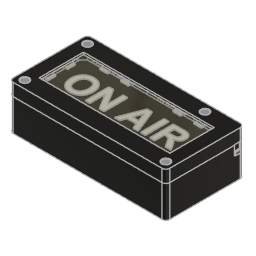
little-on-air-v2 (Autodesk Fusion 360 design; units mm, degrees)
description: Front face down; removable optics; shared left/bottom datums
description: Laser only; rear-engrave mirrored shared vector master
description: 1.6 mm black; 0.4 mm white letters; integral hidden spacer pads
description: Flat frame down, LED pads up; no electronics mounts
description: Optional 1.6 mm laminate only; omit with printed backing; print 0.1 mm layers
description: Rear face down; integral nests, ports, controls and blind M3 bosses
description: Front face down, contact legs up; use M3x8 button heads
description: Flat-sided golf tee; broad flat side down; positive 0.5 mm travel stop
description: Socket end down; 45 degree expanding shoulder; grip passes through wall
description: 52x21x10 pouch; foam and wiring not modeled
description: Provisional bare PCB, USB and component envelopes
description: 21x17.8 board; reset and populated envelopes remain provisional
description: Updated actuator dimensions; throw interpreted from slot length
description: 8x8x2; emitter offset assumed 1 mm
description: 4x25 socket head, 2x6 button head, 2x8 button head
description: Eight standard 5.5 AF x 2.4 mm nuts
Autodesk Fusion 360 part; units mm, degrees
(part 1 of 5)
sketch "Front bezel envelope profile" plane through (0, 0, 0) normal (0, 0, 1) x (1, 0, 0) in component "01 Front optical bezel"
  line L0 (3, 0) -> (117, 0)
  line L1 (120, 3) -> (120, 57)
  line L2 (117, 60) -> (3, 60)
  line L3 (0, 57) -> (0, 3)
  arc A0 (117, 0) -> (120, 3) centre (117, 3) ccw
  arc A1 (120, 57) -> (117, 60) centre (117, 57) ccw
  arc A2 (3, 60) -> (0, 57) centre (3, 57) ccw
  arc A3 (0, 3) -> (3, 0) centre (3, 3) ccw
extrude "Front bezel envelope" add sketch "Front bezel envelope profile" against normal blind 9.5 makes body 1 in component "01 Front optical bezel"
ref_plane "WorkPlane1" through (0, 0, -1.6) normal (0, 0, 1) x (1, 0, 0) in component "01 Front optical bezel"
sketch "Rear open cavity profile" plane through (0, 0, -1.6) normal (0, 0, 1) x (1, 0, 0) in component "01 Front optical bezel"
  line L0 (2.4, 2.4) -> (117.6, 2.4)
  line L1 (117.6, 2.4) -> (117.6, 57.6)
  line L2 (117.6, 57.6) -> (2.4, 57.6)
  line L3 (2.4, 57.6) -> (2.4, 2.4)
  dimension "d39" = 115.2
  dimension "d40" = 55.2
  measures "d39" horizontal distance of L0.start L0.end
  measures "d40" vertical distance of L0.end L1.end
extrude "Rear open cavity" cut sketch "Rear open cavity profile" against normal blind 8 bodies 1 in component "01 Front optical bezel"
ref_plane "WorkPlane2" through (0, 0, 0.02) normal (0, 0, 1) x (1, 0, 0) in component "01 Front optical bezel"
sketch "Visible optical window profile" plane through (0, 0, 0.02) normal (0, 0, 1) x (1, 0, 0) in component "01 Front optical bezel"
  line L0 (10, 13) -> (110, 13)
  line L1 (110, 13) -> (110, 47)
  line L2 (110, 47) -> (10, 47)
  line L3 (10, 47) -> (10, 13)
  dimension "d45" = 100
  dimension "d46" = 34
  measures "d45" horizontal distance of L0.start L0.end
  measures "d46" vertical distance of L0.end L1.end
extrude "Visible optical window" cut sketch "Visible optical window profile" against normal blind 1.64 bodies 1 in component "01 Front optical bezel"
ref_plane "WorkPlane3" through (0, 0, -1.5) normal (0, 0, 1) x (1, 0, 0) in component "01 Front optical bezel"
sketch "Front compression seat profile" plane through (0, 0, -1.5) normal (0, 0, 1) x (1, 0, 0) in component "01 Front optical bezel"
  line L0 (1.8, 1.8) -> (10.2, 1.8)
  line L1 (10.2, 1.8) -> (10.2, 10.2)
  line L2 (10.2, 10.2) -> (1.8, 10.2)
  line L3 (1.8, 10.2) -> (1.8, 1.8)
  dimension "d51" = 8.4
  dimension "d52" = 8.4
  measures "d51" horizontal distance of L0.start L0.end
  measures "d52" vertical distance of L0.end L1.end
extrude "Front compression seat" add sketch "Front compression seat profile" against normal blind 8 separate body makes body 2 in component "01 Front optical bezel"
ref_plane "WorkPlane4" through (0, 0, -1.5) normal (0, 0, 1) x (1, 0, 0) in component "01 Front optical bezel"
sketch "Front compression seat profile (1)" plane through (0, 0, -1.5) normal (0, 0, 1) x (1, 0, 0) in component "01 Front optical bezel"
  line L0 (109.8, 1.8) -> (118.2, 1.8)
  line L1 (118.2, 1.8) -> (118.2, 10.2)
  line L2 (118.2, 10.2) -> (109.8, 10.2)
  line L3 (109.8, 10.2) -> (109.8, 1.8)
  dimension "d57" = 8.4
  dimension "d58" = 8.4
  measures "d57" horizontal distance of L0.start L0.end
  measures "d58" vertical distance of L0.end L1.end
extrude "Front compression seat (1)" add sketch "Front compression seat profile (1)" against normal blind 8 separate body makes body 3 in component "01 Front optical bezel"
ref_plane "WorkPlane5" through (0, 0, -1.5) normal (0, 0, 1) x (1, 0, 0) in component "01 Front optical bezel"
sketch "Front compression seat profile (2)" plane through (0, 0, -1.5) normal (0, 0, 1) x (1, 0, 0) in component "01 Front optical bezel"
  line L0 (1.8, 49.8) -> (10.2, 49.8)
  line L1 (10.2, 49.8) -> (10.2, 58.2)
  line L2 (10.2, 58.2) -> (1.8, 58.2)
  line L3 (1.8, 58.2) -> (1.8, 49.8)
  dimension "d63" = 8.4
  dimension "d64" = 8.4
  measures "d63" horizontal distance of L0.start L0.end
  measures "d64" vertical distance of L0.end L1.end
extrude "Front compression seat (2)" add sketch "Front compression seat profile (2)" against normal blind 8 separate body makes body 4 in component "01 Front optical bezel"
ref_plane "WorkPlane6" through (0, 0, -1.5) normal (0, 0, 1) x (1, 0, 0) in component "01 Front optical bezel"
sketch "Front compression seat profile (3)" plane through (0, 0, -1.5) normal (0, 0, 1) x (1, 0, 0) in component "01 Front optical bezel"
  line L0 (91.8, 49.8) -> (100.2, 49.8)
  line L1 (100.2, 49.8) -> (100.2, 58.2)
  line L2 (100.2, 58.2) -> (91.8, 58.2)
  line L3 (91.8, 58.2) -> (91.8, 49.8)
  dimension "d69" = 8.4
  dimension "d70" = 8.4
  measures "d69" horizontal distance of L0.start L0.end
  measures "d70" vertical distance of L0.end L1.end
extrude "Front compression seat (3)" add sketch "Front compression seat profile (3)" against normal blind 8 separate body makes body 5 in component "01 Front optical bezel"
combine "Union manufactured solid" operation add target body 1 tool bodies 2 3 4 5 in component "01 Front optical bezel"
ref_plane "WorkPlane7" through (0, 0, 0.02) normal (0, 0, 1) x (1, 0, 0) in component "01 Front optical bezel"
sketch "M3 through clearance profile" plane through (0, 0, 0.02) normal (0, 0, 1) x (1, 0, 0) in component "01 Front optical bezel"
  circle A0 centre (6, 6) radius 1.7
  dimension "d75" = 3.4
  measures "d75" diameter of A0
extrude "M3 through clearance" cut sketch "M3 through clearance profile" against normal blind 9.6 bodies 1 in component "01 Front optical bezel"
ref_plane "WorkPlane8" through (0, 0, 0.02) normal (0, 0, 1) x (1, 0, 0) in component "01 Front optical bezel"
sketch "Recessed socket head profile" plane through (0, 0, 0.02) normal (0, 0, 1) x (1, 0, 0) in component "01 Front optical bezel"
  circle A0 centre (6, 6) radius 3.2
  dimension "d80" = 6.4
  measures "d80" diameter of A0
extrude "Recessed socket head" cut sketch "Recessed socket head profile" against normal blind 3.22 bodies 1 in component "01 Front optical bezel"
ref_plane "WorkPlane9" through (0, 0, 0.02) normal (0, 0, 1) x (1, 0, 0) in component "01 Front optical bezel"
sketch "M3 through clearance profile (1)" plane through (0, 0, 0.02) normal (0, 0, 1) x (1, 0, 0) in component "01 Front optical bezel"
  circle A0 centre (114, 6) radius 1.7
  dimension "d85" = 3.4
  measures "d85" diameter of A0
extrude "M3 through clearance (1)" cut sketch "M3 through clearance profile (1)" against normal blind 9.6 bodies 1 in component "01 Front optical bezel"
ref_plane "WorkPlane10" through (0, 0, 0.02) normal (0, 0, 1) x (1, 0, 0) in component "01 Front optical bezel"
sketch "Recessed socket head profile (1)" plane through (0, 0, 0.02) normal (0, 0, 1) x (1, 0, 0) in component "01 Front optical bezel"
  circle A0 centre (114, 6) radius 3.2
  dimension "d90" = 6.4
  measures "d90" diameter of A0
extrude "Recessed socket head (1)" cut sketch "Recessed socket head profile (1)" against normal blind 3.22 bodies 1 in component "01 Front optical bezel"
ref_plane "WorkPlane11" through (0, 0, 0.02) normal (0, 0, 1) x (1, 0, 0) in component "01 Front optical bezel"
sketch "M3 through clearance profile (2)" plane through (0, 0, 0.02) normal (0, 0, 1) x (1, 0, 0) in component "01 Front optical bezel"
  circle A0 centre (6, 54) radius 1.7
  dimension "d95" = 3.4
  measures "d95" diameter of A0
extrude "M3 through clearance (2)" cut sketch "M3 through clearance profile (2)" against normal blind 9.6 bodies 1 in component "01 Front optical bezel"
ref_plane "WorkPlane12" through (0, 0, 0.02) normal (0, 0, 1) x (1, 0, 0) in component "01 Front optical bezel"
sketch "Recessed socket head profile (2)" plane through (0, 0, 0.02) normal (0, 0, 1) x (1, 0, 0) in component "01 Front optical bezel"
  circle A0 centre (6, 54) radius 3.2
  dimension "d100" = 6.4
  measures "d100" diameter of A0
extrude "Recessed socket head (2)" cut sketch "Recessed socket head profile (2)" against normal blind 3.22 bodies 1 in component "01 Front optical bezel"
ref_plane "WorkPlane13" through (0, 0, 0.02) normal (0, 0, 1) x (1, 0, 0) in component "01 Front optical bezel"
sketch "M3 through clearance profile (3)" plane through (0, 0, 0.02) normal (0, 0, 1) x (1, 0, 0) in component "01 Front optical bezel"
  circle A0 centre (96, 54) radius 1.7
  dimension "d105" = 3.4
  measures "d105" diameter of A0
extrude "M3 through clearance (3)" cut sketch "M3 through clearance profile (3)" against normal blind 9.6 bodies 1 in component "01 Front optical bezel"
ref_plane "WorkPlane14" through (0, 0, 0.02) normal (0, 0, 1) x (1, 0, 0) in component "01 Front optical bezel"
sketch "Recessed socket head profile (3)" plane through (0, 0, 0.02) normal (0, 0, 1) x (1, 0, 0) in component "01 Front optical bezel"
  circle A0 centre (96, 54) radius 3.2
  dimension "d110" = 6.4
  measures "d110" diameter of A0
extrude "Recessed socket head (3)" cut sketch "Recessed socket head profile (3)" against normal blind 3.22 bodies 1 in component "01 Front optical bezel"
ref_plane "WorkPlane15" through (0, 0, -1.5) normal (0, 0, 1) x (1, 0, 0) in component "01 Front optical bezel"
sketch "LED floor profile" plane through (0, 0, -1.5) normal (0, 0, 1) x (1, 0, 0) in component "01 Front optical bezel"
  line L0 (35.7, 2.4) -> (44.3, 2.4)
  line L1 (44.3, 2.4) -> (44.3, 11.2)
  line L2 (44.3, 11.2) -> (35.7, 11.2)
  line L3 (35.7, 11.2) -> (35.7, 2.4)
  dimension "d115" = 8.6
  dimension "d116" = 8.8
  measures "d115" horizontal distance of L0.start L0.end
  measures "d116" vertical distance of L0.end L1.end
extrude "LED floor" add sketch "LED floor profile" against normal blind 0.6875 separate body makes body 6 in component "01 Front optical bezel"
ref_plane "WorkPlane16" through (0, 0, -1.5) normal (0, 0, 1) x (1, 0, 0) in component "01 Front optical bezel"
sketch "LED lateral guide profile" plane through (0, 0, -1.5) normal (0, 0, 1) x (1, 0, 0) in component "01 Front optical bezel"
  line L0 (34.5, 2.4) -> (35.75, 2.4)
  line L1 (35.75, 2.4) -> (35.75, 11.2)
  line L2 (35.75, 11.2) -> (34.5, 11.2)
  line L3 (34.5, 11.2) -> (34.5, 2.4)
  dimension "d121" = 1.25
  dimension "d122" = 8.8
  measures "d121" horizontal distance of L0.start L0.end
  measures "d122" vertical distance of L0.end L1.end
extrude "LED lateral guide" add sketch "LED lateral guide profile" against normal blind 3 separate body makes body 7 in component "01 Front optical bezel"
ref_plane "WorkPlane17" through (0, 0, -1.5) normal (0, 0, 1) x (1, 0, 0) in component "01 Front optical bezel"
sketch "LED lateral guide profile (1)" plane through (0, 0, -1.5) normal (0, 0, 1) x (1, 0, 0) in component "01 Front optical bezel"
  line L0 (44.25, 2.4) -> (45.5, 2.4)
  line L1 (45.5, 2.4) -> (45.5, 11.2)
  line L2 (45.5, 11.2) -> (44.25, 11.2)
  line L3 (44.25, 11.2) -> (44.25, 2.4)
  dimension "d127" = 1.25
  dimension "d128" = 8.8
  measures "d127" horizontal distance of L0.start L0.end
  measures "d128" vertical distance of L0.end L1.end
extrude "LED lateral guide (1)" add sketch "LED lateral guide profile (1)" against normal blind 3 separate body makes body 8 in component "01 Front optical bezel"
ref_plane "WorkPlane18" through (0, 0, -1.5) normal (0, 0, 1) x (1, 0, 0) in component "01 Front optical bezel"
sketch "LED floor profile (1)" plane through (0, 0, -1.5) normal (0, 0, 1) x (1, 0, 0) in component "01 Front optical bezel"
  line L0 (35.7, 48.8) -> (44.3, 48.8)
  line L1 (44.3, 48.8) -> (44.3, 57.6)
  line L2 (44.3, 57.6) -> (35.7, 57.6)
  line L3 (35.7, 57.6) -> (35.7, 48.8)
  dimension "d133" = 8.6
  dimension "d134" = 8.8
  measures "d133" horizontal distance of L0.start L0.end
  measures "d134" vertical distance of L0.end L1.end
extrude "LED floor (1)" add sketch "LED floor profile (1)" against normal blind 0.6875 separate body makes body 9 in component "01 Front optical bezel"
ref_plane "WorkPlane19" through (0, 0, -1.5) normal (0, 0, 1) x (1, 0, 0) in component "01 Front optical bezel"
sketch "LED lateral guide profile (2)" plane through (0, 0, -1.5) normal (0, 0, 1) x (1, 0, 0) in component "01 Front optical bezel"
  line L0 (34.5, 48.8) -> (35.75, 48.8)
  line L1 (35.75, 48.8) -> (35.75, 57.6)
  line L2 (35.75, 57.6) -> (34.5, 57.6)
  line L3 (34.5, 57.6) -> (34.5, 48.8)
  dimension "d139" = 1.25
  dimension "d140" = 8.8
  measures "d139" horizontal distance of L0.start L0.end
  measures "d140" vertical distance of L0.end L1.end
extrude "LED lateral guide (2)" add sketch "LED lateral guide profile (2)" against normal blind 3 separate body makes body 10 in component "01 Front optical bezel"
ref_plane "WorkPlane20" through (0, 0, -1.5) normal (0, 0, 1) x (1, 0, 0) in component "01 Front optical bezel"
sketch "LED lateral guide profile (3)" plane through (0, 0, -1.5) normal (0, 0, 1) x (1, 0, 0) in component "01 Front optical bezel"
  line L0 (44.25, 48.8) -> (45.5, 48.8)
  line L1 (45.5, 48.8) -> (45.5, 57.6)
  line L2 (45.5, 57.6) -> (44.25, 57.6)
  line L3 (44.25, 57.6) -> (44.25, 48.8)
  dimension "d145" = 1.25
  dimension "d146" = 8.8
  measures "d145" horizontal distance of L0.start L0.end
  measures "d146" vertical distance of L0.end L1.end
extrude "LED lateral guide (3)" add sketch "LED lateral guide profile (3)" against normal blind 3 separate body makes body 11 in component "01 Front optical bezel"
ref_plane "WorkPlane21" through (0, 0, -1.5) normal (0, 0, 1) x (1, 0, 0) in component "01 Front optical bezel"
sketch "LED floor profile (2)" plane through (0, 0, -1.5) normal (0, 0, 1) x (1, 0, 0) in component "01 Front optical bezel"
  line L0 (75.7, 2.4) -> (84.3, 2.4)
  line L1 (84.3, 2.4) -> (84.3, 11.2)
  line L2 (84.3, 11.2) -> (75.7, 11.2)
  line L3 (75.7, 11.2) -> (75.7, 2.4)
  dimension "d151" = 8.6
  dimension "d152" = 8.8
  measures "d151" horizontal distance of L0.start L0.end
  measures "d152" vertical distance of L0.end L1.end
extrude "LED floor (2)" add sketch "LED floor profile (2)" against normal blind 0.6875 separate body makes body 12 in component "01 Front optical bezel"
ref_plane "WorkPlane22" through (0, 0, -1.5) normal (0, 0, 1) x (1, 0, 0) in component "01 Front optical bezel"
sketch "LED lateral guide profile (4)" plane through (0, 0, -1.5) normal (0, 0, 1) x (1, 0, 0) in component "01 Front optical bezel"
  line L0 (74.5, 2.4) -> (75.75, 2.4)
  line L1 (75.75, 2.4) -> (75.75, 11.2)
  line L2 (75.75, 11.2) -> (74.5, 11.2)
  line L3 (74.5, 11.2) -> (74.5, 2.4)
  dimension "d157" = 1.25
  dimension "d158" = 8.8
  measures "d157" horizontal distance of L0.start L0.end
  measures "d158" vertical distance of L0.end L1.end
extrude "LED lateral guide (4)" add sketch "LED lateral guide profile (4)" against normal blind 3 separate body makes body 13 in component "01 Front optical bezel"
ref_plane "WorkPlane23" through (0, 0, -1.5) normal (0, 0, 1) x (1, 0, 0) in component "01 Front optical bezel"
sketch "LED lateral guide profile (5)" plane through (0, 0, -1.5) normal (0, 0, 1) x (1, 0, 0) in component "01 Front optical bezel"
  line L0 (84.25, 2.4) -> (85.5, 2.4)
  line L1 (85.5, 2.4) -> (85.5, 11.2)
  line L2 (85.5, 11.2) -> (84.25, 11.2)
  line L3 (84.25, 11.2) -> (84.25, 2.4)
  dimension "d163" = 1.25
  dimension "d164" = 8.8
  measures "d163" horizontal distance of L0.start L0.end
  measures "d164" vertical distance of L0.end L1.end
extrude "LED lateral guide (5)" add sketch "LED lateral guide profile (5)" against normal blind 3 separate body makes body 14 in component "01 Front optical bezel"
ref_plane "WorkPlane24" through (0, 0, -1.5) normal (0, 0, 1) x (1, 0, 0) in component "01 Front optical bezel"
sketch "LED floor profile (3)" plane through (0, 0, -1.5) normal (0, 0, 1) x (1, 0, 0) in component "01 Front optical bezel"
  line L0 (75.7, 48.8) -> (84.3, 48.8)
  line L1 (84.3, 48.8) -> (84.3, 57.6)
  line L2 (84.3, 57.6) -> (75.7, 57.6)
  line L3 (75.7, 57.6) -> (75.7, 48.8)
  dimension "d169" = 8.6
  dimension "d170" = 8.8
  measures "d169" horizontal distance of L0.start L0.end
  measures "d170" vertical distance of L0.end L1.end
extrude "LED floor (3)" add sketch "LED floor profile (3)" against normal blind 0.6875 separate body makes body 15 in component "01 Front optical bezel"
ref_plane "WorkPlane25" through (0, 0, -1.5) normal (0, 0, 1) x (1, 0, 0) in component "01 Front optical bezel"
sketch "LED lateral guide profile (6)" plane through (0, 0, -1.5) normal (0, 0, 1) x (1, 0, 0) in component "01 Front optical bezel"
  line L0 (74.5, 48.8) -> (75.75, 48.8)
  line L1 (75.75, 48.8) -> (75.75, 57.6)
  line L2 (75.75, 57.6) -> (74.5, 57.6)
  line L3 (74.5, 57.6) -> (74.5, 48.8)
  dimension "d175" = 1.25
  dimension "d176" = 8.8
  measures "d175" horizontal distance of L0.start L0.end
  measures "d176" vertical distance of L0.end L1.end
extrude "LED lateral guide (6)" add sketch "LED lateral guide profile (6)" against normal blind 3 separate body makes body 16 in component "01 Front optical bezel"
ref_plane "WorkPlane26" through (0, 0, -1.5) normal (0, 0, 1) x (1, 0, 0) in component "01 Front optical bezel"
sketch "LED lateral guide profile (7)" plane through (0, 0, -1.5) normal (0, 0, 1) x (1, 0, 0) in component "01 Front optical bezel"
  line L0 (84.25, 48.8) -> (85.5, 48.8)
  line L1 (85.5, 48.8) -> (85.5, 57.6)
  line L2 (85.5, 57.6) -> (84.25, 57.6)
  line L3 (84.25, 57.6) -> (84.25, 48.8)
  dimension "d181" = 1.25
  dimension "d182" = 8.8
  measures "d181" horizontal distance of L0.start L0.end
  measures "d182" vertical distance of L0.end L1.end
extrude "LED lateral guide (7)" add sketch "LED lateral guide profile (7)" against normal blind 3 separate body makes body 17 in component "01 Front optical bezel"
ref_plane "WorkPlane27" through (0, 0, -1.5) normal (0, 0, 1) x (1, 0, 0) in component "01 Front optical bezel"
sketch "Shared left datum profile" plane through (0, 0, -1.5) normal (0, 0, 1) x (1, 0, 0) in component "01 Front optical bezel"
  line L0 (6.5, 20) -> (8, 20)
  line L1 (8, 20) -> (8, 26)
  line L2 (8, 26) -> (6.5, 26)
  line L3 (6.5, 26) -> (6.5, 20)
  dimension "d187" = 1.5
  dimension "d188" = 6
  measures "d187" horizontal distance of L0.start L0.end
  measures "d188" vertical distance of L0.end L1.end
extrude "Shared left datum" add sketch "Shared left datum profile" against normal blind 5.775 separate body makes body 18 in component "01 Front optical bezel"
ref_plane "WorkPlane28" through (0, 0, -1.5) normal (0, 0, 1) x (1, 0, 0) in component "01 Front optical bezel"
sketch "Shared left datum profile (1)" plane through (0, 0, -1.5) normal (0, 0, 1) x (1, 0, 0) in component "01 Front optical bezel"
  line L0 (6.5, 35) -> (8, 35)
  line L1 (8, 35) -> (8, 41)
  line L2 (8, 41) -> (6.5, 41)
  line L3 (6.5, 41) -> (6.5, 35)
  dimension "d193" = 1.5
  dimension "d194" = 6
  measures "d193" horizontal distance of L0.start L0.end
  measures "d194" vertical distance of L0.end L1.end
extrude "Shared left datum (1)" add sketch "Shared left datum profile (1)" against normal blind 5.775 separate body makes body 19 in component "01 Front optical bezel"
ref_plane "WorkPlane29" through (0, 0, -1.5) normal (0, 0, 1) x (1, 0, 0) in component "01 Front optical bezel"
sketch "Shared lower datum profile" plane through (0, 0, -1.5) normal (0, 0, 1) x (1, 0, 0) in component "01 Front optical bezel"
  line L0 (22, 9.5) -> (28, 9.5)
  line L1 (28, 9.5) -> (28, 11)
  line L2 (28, 11) -> (22, 11)
  line L3 (22, 11) -> (22, 9.5)
  dimension "d199" = 6
  dimension "d200" = 1.5
  measures "d199" horizontal distance of L0.start L0.end
  measures "d200" vertical distance of L0.end L1.end
extrude "Shared lower datum" add sketch "Shared lower datum profile" against normal blind 5.775 separate body makes body 20 in component "01 Front optical bezel"
ref_plane "WorkPlane30" through (0, 0, -1.5) normal (0, 0, 1) x (1, 0, 0) in component "01 Front optical bezel"
sketch "Shared lower datum profile (1)" plane through (0, 0, -1.5) normal (0, 0, 1) x (1, 0, 0) in component "01 Front optical bezel"
  line L0 (94, 9.5) -> (100, 9.5)
  line L1 (100, 9.5) -> (100, 11)
  line L2 (100, 11) -> (94, 11)
  line L3 (94, 11) -> (94, 9.5)
  dimension "d205" = 6
  dimension "d206" = 1.5
  measures "d205" horizontal distance of L0.start L0.end
  measures "d206" vertical distance of L0.end L1.end
extrude "Shared lower datum (1)" add sketch "Shared lower datum profile (1)" against normal blind 5.775 separate body makes body 21 in component "01 Front optical bezel"
ref_plane "WorkPlane31" through (0, 0, -1.5) normal (0, 0, 1) x (1, 0, 0) in component "01 Front optical bezel"
sketch "Right compliant pad wall profile" plane through (0, 0, -1.5) normal (0, 0, 1) x (1, 0, 0) in component "01 Front optical bezel"
  line L0 (112.5, 20) -> (114.1, 20)
  line L1 (114.1, 20) -> (114.1, 26)
  line L2 (114.1, 26) -> (112.5, 26)
  line L3 (112.5, 26) -> (112.5, 20)
  dimension "d211" = 1.6
  dimension "d212" = 6
  measures "d211" horizontal distance of L0.start L0.end
  measures "d212" vertical distance of L0.end L1.end
extrude "Right compliant pad wall" add sketch "Right compliant pad wall profile" against normal blind 5.775 separate body makes body 22 in component "01 Front optical bezel"
ref_plane "WorkPlane32" through (0, 0, -1.5) normal (0, 0, 1) x (1, 0, 0) in component "01 Front optical bezel"
sketch "Right compliant pad wall profile (1)" plane through (0, 0, -1.5) normal (0, 0, 1) x (1, 0, 0) in component "01 Front optical bezel"
  line L0 (112.5, 35) -> (114.1, 35)
  line L1 (114.1, 35) -> (114.1, 41)
  line L2 (114.1, 41) -> (112.5, 41)
  line L3 (112.5, 41) -> (112.5, 35)
  dimension "d217" = 1.6
  dimension "d218" = 6
  measures "d217" horizontal distance of L0.start L0.end
  measures "d218" vertical distance of L0.end L1.end
extrude "Right compliant pad wall (1)" add sketch "Right compliant pad wall profile (1)" against normal blind 5.775 separate body makes body 23 in component "01 Front optical bezel"
ref_plane "WorkPlane33" through (0, 0, -1.5) normal (0, 0, 1) x (1, 0, 0) in component "01 Front optical bezel"
sketch "Upper compliant pad wall profile" plane through (0, 0, -1.5) normal (0, 0, 1) x (1, 0, 0) in component "01 Front optical bezel"
  line L0 (22, 49.5) -> (28, 49.5)
  line L1 (28, 49.5) -> (28, 51.1)
  line L2 (28, 51.1) -> (22, 51.1)
  line L3 (22, 51.1) -> (22, 49.5)
  dimension "d223" = 6
  dimension "d224" = 1.6
  measures "d223" horizontal distance of L0.start L0.end
  measures "d224" vertical distance of L0.end L1.end
extrude "Upper compliant pad wall" add sketch "Upper compliant pad wall profile" against normal blind 5.775 separate body makes body 24 in component "01 Front optical bezel"
ref_plane "WorkPlane34" through (0, 0, -1.5) normal (0, 0, 1) x (1, 0, 0) in component "01 Front optical bezel"
sketch "Upper compliant pad wall profile (1)" plane through (0, 0, -1.5) normal (0, 0, 1) x (1, 0, 0) in component "01 Front optical bezel"
  line L0 (94, 49.5) -> (100, 49.5)
  line L1 (100, 49.5) -> (100, 51.1)
  line L2 (100, 51.1) -> (94, 51.1)
  line L3 (94, 51.1) -> (94, 49.5)
  dimension "d229" = 6
  dimension "d230" = 1.6
  measures "d229" horizontal distance of L0.start L0.end
  measures "d230" vertical distance of L0.end L1.end
extrude "Upper compliant pad wall (1)" add sketch "Upper compliant pad wall profile (1)" against normal blind 5.775 separate body makes body 25 in component "01 Front optical bezel"
ref_plane "WorkPlane35" through (0, 0, -9.1) normal (0, 0, 1) x (1, 0, 0) in component "01 Front optical bezel"
sketch "Side tongue root profile" plane through (0, 0, -9.1) normal (0, 0, 1) x (1, 0, 0) in component "01 Front optical bezel"
  line L0 (2.3, 17) -> (3.85, 17)
  line L1 (3.85, 17) -> (3.85, 26)
  line L2 (3.85, 26) -> (2.3, 26)
  line L3 (2.3, 26) -> (2.3, 17)
  dimension "d235" = 1.55
  dimension "d236" = 9
  measures "d235" horizontal distance of L0.start L0.end
  measures "d236" vertical distance of L0.end L1.end
extrude "Side tongue root" add sketch "Side tongue root profile" against normal blind 0.4 separate body makes body 26 in component "01 Front optical bezel"
ref_plane "WorkPlane36" through (0, 0, -9.1) normal (0, 0, 1) x (1, 0, 0) in component "01 Front optical bezel"
sketch "Side tongue root profile (1)" plane through (0, 0, -9.1) normal (0, 0, 1) x (1, 0, 0) in component "01 Front optical bezel"
  line L0 (116.15, 17) -> (117.7, 17)
  line L1 (117.7, 17) -> (117.7, 26)
  line L2 (117.7, 26) -> (116.15, 26)
  line L3 (116.15, 26) -> (116.15, 17)
  dimension "d241" = 1.55
  dimension "d242" = 9
  measures "d241" horizontal distance of L0.start L0.end
  measures "d242" vertical distance of L0.end L1.end
extrude "Side tongue root (1)" add sketch "Side tongue root profile (1)" against normal blind 0.4 separate body makes body 27 in component "01 Front optical bezel"
ref_plane "WorkPlane37" through (0, 0, -9.3) normal (0, 0, 1) x (1, 0, 0) in component "01 Front optical bezel"
sketch "Side locating tongue profile" plane through (0, 0, -9.3) normal (0, 0, 1) x (1, 0, 0) in component "01 Front optical bezel"
  line L0 (2.65, 17) -> (3.85, 17)
  line L1 (3.85, 17) -> (3.85, 26)
  line L2 (3.85, 26) -> (2.65, 26)
  line L3 (2.65, 26) -> (2.65, 17)
  dimension "d247" = 1.2
  dimension "d248" = 9
  measures "d247" horizontal distance of L0.start L0.end
  measures "d248" vertical distance of L0.end L1.end
extrude "Side locating tongue" add sketch "Side locating tongue profile" against normal blind 1.7 separate body makes body 28 in component "01 Front optical bezel"
ref_plane "WorkPlane38" through (0, 0, -9.3) normal (0, 0, 1) x (1, 0, 0) in component "01 Front optical bezel"
sketch "Side locating tongue profile (1)" plane through (0, 0, -9.3) normal (0, 0, 1) x (1, 0, 0) in component "01 Front optical bezel"
  line L0 (116.15, 17) -> (117.35, 17)
  line L1 (117.35, 17) -> (117.35, 26)
  line L2 (117.35, 26) -> (116.15, 26)
  line L3 (116.15, 26) -> (116.15, 17)
  dimension "d253" = 1.2
  dimension "d254" = 9
  measures "d253" horizontal distance of L0.start L0.end
  measures "d254" vertical distance of L0.end L1.end
extrude "Side locating tongue (1)" add sketch "Side locating tongue profile (1)" against normal blind 1.7 separate body makes body 29 in component "01 Front optical bezel"
ref_plane "WorkPlane39" through (0, 0, -9.1) normal (0, 0, 1) x (1, 0, 0) in component "01 Front optical bezel"
sketch "Upper tongue root profile" plane through (0, 0, -9.1) normal (0, 0, 1) x (1, 0, 0) in component "01 Front optical bezel"
  line L0 (36, 56.15) -> (46, 56.15)
  line L1 (46, 56.15) -> (46, 57.7)
  line L2 (46, 57.7) -> (36, 57.7)
  line L3 (36, 57.7) -> (36, 56.15)
  dimension "d259" = 10
  dimension "d260" = 1.55
  measures "d259" horizontal distance of L0.start L0.end
  measures "d260" vertical distance of L0.end L1.end
extrude "Upper tongue root" add sketch "Upper tongue root profile" against normal blind 0.4 separate body makes body 30 in component "01 Front optical bezel"
ref_plane "WorkPlane40" through (0, 0, -9.3) normal (0, 0, 1) x (1, 0, 0) in component "01 Front optical bezel"
sketch "Upper locating tongue profile" plane through (0, 0, -9.3) normal (0, 0, 1) x (1, 0, 0) in component "01 Front optical bezel"
  line L0 (36, 56.15) -> (46, 56.15)
  line L1 (46, 56.15) -> (46, 57.35)
  line L2 (46, 57.35) -> (36, 57.35)
  line L3 (36, 57.35) -> (36, 56.15)
  dimension "d265" = 10
  dimension "d266" = 1.2
  measures "d265" horizontal distance of L0.start L0.end
  measures "d266" vertical distance of L0.end L1.end
extrude "Upper locating tongue" add sketch "Upper locating tongue profile" against normal blind 1.7 separate body makes body 31 in component "01 Front optical bezel"
combine "Union manufactured solid (1)" operation add target body 1 tool bodies 6 7 8 9 10 11 12 13 14 15 16 17 18 19 20 21 22 23 24 25 26 27 28 29 30 31 in component "01 Front optical bezel"
ref_plane "WorkPlane41" through (0, 0, -1.5) normal (0, 0, 1) x (1, 0, 0) in component "01 Front optical bezel"
sketch "Optical clamp boss profile" plane through (0, 0, -1.5) normal (0, 0, 1) x (1, 0, 0) in component "01 Front optical bezel"
  line L0 (55.8, 1.8) -> (64.2, 1.8)
  line L1 (64.2, 1.8) -> (64.2, 10.2)
  line L2 (64.2, 10.2) -> (55.8, 10.2)
  line L3 (55.8, 10.2) -> (55.8, 1.8)
  dimension "d271" = 8.4
  dimension "d272" = 8.4
  measures "d271" horizontal distance of L0.start L0.end
  measures "d272" vertical distance of L0.end L1.end
extrude "Optical clamp boss" add sketch "Optical clamp boss profile" against normal blind 5.975 separate body makes body 32 in component "01 Front optical bezel"
ref_plane "WorkPlane42" through (0, 0, -1.5) normal (0, 0, 1) x (1, 0, 0) in component "01 Front optical bezel"
sketch "Optical clamp boss profile (1)" plane through (0, 0, -1.5) normal (0, 0, 1) x (1, 0, 0) in component "01 Front optical bezel"
  line L0 (55.8, 49.8) -> (64.2, 49.8)
  line L1 (64.2, 49.8) -> (64.2, 58.2)
  line L2 (64.2, 58.2) -> (55.8, 58.2)
  line L3 (55.8, 58.2) -> (55.8, 49.8)
  dimension "d277" = 8.4
  dimension "d278" = 8.4
  measures "d277" horizontal distance of L0.start L0.end
  measures "d278" vertical distance of L0.end L1.end
extrude "Optical clamp boss (1)" add sketch "Optical clamp boss profile (1)" against normal blind 5.975 separate body makes body 33 in component "01 Front optical bezel"
combine "Union manufactured solid (2)" operation add target body 1 tool bodies 32 33 in component "01 Front optical bezel"
ref_plane "WorkPlane43" through (0, 0, -3.2) normal (0, 0, 1) x (1, 0, 0) in component "01 Front optical bezel"
sketch "Optical M3 nut trap" plane through (0, 0, -3.2) normal (0, 0, 1) x (1, 0, 0) in component "01 Front optical bezel"
  line L0 (63.3486, 6) -> (61.6743, 8.9)
  line L1 (61.6743, 8.9) -> (58.3257, 8.9)
  line L2 (58.3257, 8.9) -> (56.6514, 6)
  line L3 (56.6514, 6) -> (58.3257, 3.1)
  line L4 (58.3257, 3.1) -> (61.6743, 3.1)
  line L5 (61.6743, 3.1) -> (63.3486, 6)
extrude "Optical M3 nut trap (1)" cut sketch "Optical M3 nut trap" against normal blind 2.6 bodies 1 in component "01 Front optical bezel"
ref_plane "WorkPlane44" through (0, 0, -3.2) normal (0, 0, 1) x (1, 0, 0) in component "01 Front optical bezel"
sketch "Optical nut side entry profile" plane through (0, 0, -3.2) normal (0, 0, 1) x (1, 0, 0) in component "01 Front optical bezel"
  line L0 (60, 3.1) -> (64.5, 3.1)
  line L1 (64.5, 3.1) -> (64.5, 8.9)
  line L2 (64.5, 8.9) -> (60, 8.9)
  line L3 (60, 8.9) -> (60, 3.1)
  dimension "d287" = 4.5
  dimension "d288" = 5.8
  measures "d287" horizontal distance of L0.start L0.end
  measures "d288" vertical distance of L0.end L1.end
extrude "Optical nut side entry" cut sketch "Optical nut side entry profile" against normal blind 2.6 bodies 1 in component "01 Front optical bezel"
ref_plane "WorkPlane45" through (0, 0, -2.6) normal (0, 0, 1) x (1, 0, 0) in component "01 Front optical bezel"
sketch "Optical blind screw bore profile" plane through (0, 0, -2.6) normal (0, 0, 1) x (1, 0, 0) in component "01 Front optical bezel"
  circle A0 centre (60, 6) radius 1.7
  dimension "d293" = 3.4
  measures "d293" diameter of A0
extrude "Optical blind screw bore" cut sketch "Optical blind screw bore profile" against normal blind 4.895 bodies 1 in component "01 Front optical bezel"
ref_plane "WorkPlane46" through (0, 0, -3.2) normal (0, 0, 1) x (1, 0, 0) in component "01 Front optical bezel"
sketch "Optical M3 nut trap (1)" plane through (0, 0, -3.2) normal (0, 0, 1) x (1, 0, 0) in component "01 Front optical bezel"
  line L0 (63.3486, 54) -> (61.6743, 56.9)
  line L1 (61.6743, 56.9) -> (58.3257, 56.9)
  line L2 (58.3257, 56.9) -> (56.6514, 54)
  line L3 (56.6514, 54) -> (58.3257, 51.1)
  line L4 (58.3257, 51.1) -> (61.6743, 51.1)
  line L5 (61.6743, 51.1) -> (63.3486, 54)
extrude "Optical M3 nut trap (2)" cut sketch "Optical M3 nut trap (1)" against normal blind 2.6 bodies 1 in component "01 Front optical bezel"
ref_plane "WorkPlane47" through (0, 0, -3.2) normal (0, 0, 1) x (1, 0, 0) in component "01 Front optical bezel"
sketch "Optical nut side entry profile (1)" plane through (0, 0, -3.2) normal (0, 0, 1) x (1, 0, 0) in component "01 Front optical bezel"
  line L0 (60, 51.1) -> (64.5, 51.1)
  line L1 (64.5, 51.1) -> (64.5, 56.9)
  line L2 (64.5, 56.9) -> (60, 56.9)
  line L3 (60, 56.9) -> (60, 51.1)
  dimension "d302" = 4.5
  dimension "d303" = 5.8
  measures "d302" horizontal distance of L0.start L0.end
  measures "d303" vertical distance of L0.end L1.end
extrude "Optical nut side entry (1)" cut sketch "Optical nut side entry profile (1)" against normal blind 2.6 bodies 1 in component "01 Front optical bezel"
ref_plane "WorkPlane48" through (0, 0, -2.6) normal (0, 0, 1) x (1, 0, 0) in component "01 Front optical bezel"
sketch "Optical blind screw bore profile (1)" plane through (0, 0, -2.6) normal (0, 0, 1) x (1, 0, 0) in component "01 Front optical bezel"
  circle A0 centre (60, 54) radius 1.7
  dimension "d308" = 3.4
  measures "d308" diameter of A0
extrude "Optical blind screw bore (1)" cut sketch "Optical blind screw bore profile (1)" against normal blind 4.895 bodies 1 in component "01 Front optical bezel"
ref_plane "WorkPlane49" through (0, 0, -1.6) normal (0, 0, 1) x (1, 0, 0) in component "01 Front optical bezel"
sketch "Acrylic edge admission profile" plane through (0, 0, -1.6) normal (0, 0, 1) x (1, 0, 0) in component "01 Front optical bezel"
  line L0 (34.4, 10.75) -> (45.6, 10.75)
  line L1 (45.6, 10.75) -> (45.6, 11.2)
  line L2 (45.6, 11.2) -> (34.4, 11.2)
  line L3 (34.4, 11.2) -> (34.4, 10.75)
  dimension "d313" = 11.2
  dimension "d314" = 0.45
  measures "d313" horizontal distance of L0.start L0.end
  measures "d314" vertical distance of L0.end L1.end
extrude "Acrylic edge admission" cut sketch "Acrylic edge admission profile" against normal blind 3.7 bodies 1 in component "01 Front optical bezel"
ref_plane "WorkPlane50" through (0, 0, -1.6) normal (0, 0, 1) x (1, 0, 0) in component "01 Front optical bezel"
sketch "Acrylic edge admission profile (1)" plane through (0, 0, -1.6) normal (0, 0, 1) x (1, 0, 0) in component "01 Front optical bezel"
  line L0 (34.4, 48.8) -> (45.6, 48.8)
  line L1 (45.6, 48.8) -> (45.6, 49.25)
  line L2 (45.6, 49.25) -> (34.4, 49.25)
  line L3 (34.4, 49.25) -> (34.4, 48.8)
  dimension "d319" = 11.2
  dimension "d320" = 0.45
  measures "d319" horizontal distance of L0.start L0.end
  measures "d320" vertical distance of L0.end L1.end
extrude "Acrylic edge admission (1)" cut sketch "Acrylic edge admission profile (1)" against normal blind 3.7 bodies 1 in component "01 Front optical bezel"
ref_plane "WorkPlane51" through (0, 0, -1.6) normal (0, 0, 1) x (1, 0, 0) in component "01 Front optical bezel"
sketch "Acrylic edge admission profile (2)" plane through (0, 0, -1.6) normal (0, 0, 1) x (1, 0, 0) in component "01 Front optical bezel"
  line L0 (74.4, 10.75) -> (85.6, 10.75)
  line L1 (85.6, 10.75) -> (85.6, 11.2)
  line L2 (85.6, 11.2) -> (74.4, 11.2)
  line L3 (74.4, 11.2) -> (74.4, 10.75)
  dimension "d325" = 11.2
  dimension "d326" = 0.45
  measures "d325" horizontal distance of L0.start L0.end
  measures "d326" vertical distance of L0.end L1.end
extrude "Acrylic edge admission (2)" cut sketch "Acrylic edge admission profile (2)" against normal blind 3.7 bodies 1 in component "01 Front optical bezel"
ref_plane "WorkPlane52" through (0, 0, -1.6) normal (0, 0, 1) x (1, 0, 0) in component "01 Front optical bezel"
sketch "Acrylic edge admission profile (3)" plane through (0, 0, -1.6) normal (0, 0, 1) x (1, 0, 0) in component "01 Front optical bezel"
  line L0 (74.4, 48.8) -> (85.6, 48.8)
  line L1 (85.6, 48.8) -> (85.6, 49.25)
  line L2 (85.6, 49.25) -> (74.4, 49.25)
  line L3 (74.4, 49.25) -> (74.4, 48.8)
  dimension "d331" = 11.2
  dimension "d332" = 0.45
  measures "d331" horizontal distance of L0.start L0.end
  measures "d332" vertical distance of L0.end L1.end
extrude "Acrylic edge admission (3)" cut sketch "Acrylic edge admission profile (3)" against normal blind 3.7 bodies 1 in component "01 Front optical bezel"
ref_plane "WorkPlane1" through (0, 0, -1.6) normal (0, 0, 1) x (1, 0, 0) in component "02 Clear acrylic"
sketch "Keyed acrylic outline" plane through (0, 0, -1.6) normal (0, 0, 1) x (1, 0, 0) in component "02 Clear acrylic"
  line L0 (8, 11) -> (112, 11)
  line L1 (112, 11) -> (112, 49)
  line L2 (112, 49) -> (11, 49)
  line L3 (11, 49) -> (8, 46)
  line L4 (8, 46) -> (8, 11)
extrude "Clear acrylic sheet" add sketch "Keyed acrylic outline" against normal blind 3.175 separate body makes body 34 in component "02 Clear acrylic"
ref_plane "WorkPlane2" through (0, 0, -4.775) normal (0, 0, 1) x (1, 0, 0) in component "02 Clear acrylic"